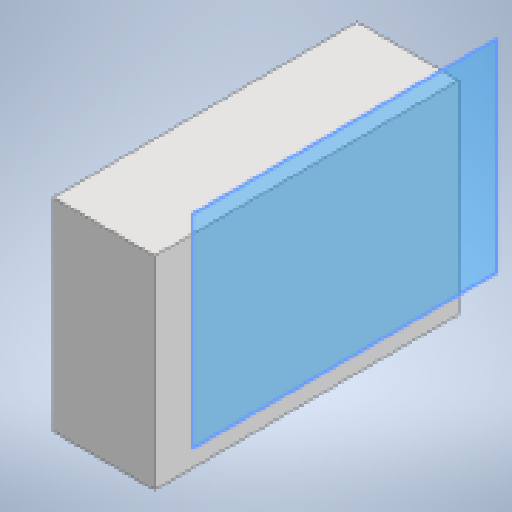
# Autodesk Inventor part: BSH 03 upstairs
Saved by Autodesk Inventor 2025 (Build 290162010, 162A)
## iProperties
Created: 2024-08-27
Part Number: BSH 03 upstairs
Material: Generic
Document SubType Name: Modeling
Designer: DELL
Density: 1 g/cm^3
Appearance: Default
Author: DELL
Autodesk Inventor part; units mm, degrees
ref_plane "YZ Plane" through (0, 0, 0) normal (1, 0, 0) x (0, 1, 0)
ref_plane "XZ Plane" through (0, 0, 0) normal (0, 1, 0) x (-1, 0, 0)
ref_plane "XY Plane" through (0, 0, 0) normal (0, 0, 1) x (1, 0, 0)
sketch "Sketch1" plane through (0, 0, 0) normal (0, 0, 1) x (1, 0, 0)
  line L0 (500, 1500) -> (-500, 1500)
  line L1 (-500, 1500) -> (-500, -1500)
  line L2 (-500, -1500) -> (500, -1500)
  line L3 (500, -1500) -> (500, 1500)
  line L4 (500, 1500) -> (-500, -1500) construction
  line L5 (-500, 1500) -> (500, -1500) construction
  point P0 (0, 0)
  dimension "d0" = 1000
  dimension "d1" = 3000
  constraints: 12 end point, 2 midpoint, 2 parallel, 1 horizontal, 1 perpendicular
  measures "d0" distance of L2.end L1.end
  measures "d1" distance of L1.end L0.end
extrude "Extrusion1" add sketch "Sketch1" along normal blind 2000
sketch "Sketch2" plane through (-500, -1500, 0) normal (-1, 0, 0) x (0, 0, 1)
  line L0 (0, 3000) -> (0, 0) projected
  line L1 (0, 0) -> (2000, 0) projected
  line L2 (2000, 3000) -> (2000, 0) projected
  line L3 (0, 3000) -> (2000, 3000) projected
  line L4 (1800, 0) -> (1800, -250)
  line L5 (1800, -250) -> (1600, -250)
  line L6 (1600, -250) -> (1800, 0)
  point P0 (0, 1500)
  dimension "d4" = 250
  dimension "d5" = 200
  dimension "d6" = 200
  dimension "d7" = 51.34
  constraints: 6 end point, 1 perpendicular, 1 point on line, 1 vertical
  measures "d4" distance of L4.start L4.end
  measures "d5" distance of L4.end L5.end
  measures "d6" distance between parallel lines of L4 L2
  measures "d7" angle of L1 L6
extrude "Extrusion2" add sketch "Sketch2" against normal up to surface (1000 mm away) contours L4 L5 L6
pattern_linear "Rectangular Pattern1" count 9 spacing 320 along (0, -0.7808688, -0.624695) of "Extrusion2"
equation "\"d6\" = d5"
body "Solid1"
